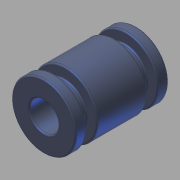
# Autodesk Inventor part: Damper
Saved by Autodesk Inventor 2011 SP2 (Build 150309200, 309)
## iProperties
Created: 2015-02-19
Part Number: Damper
Document SubType Name: Modeling
Designer: Greg Pavlik
Density: 1 g/cm^3
Author: Greg Pavlik
Autodesk Inventor part; units mm, degrees
ref_plane "YZ Plane" through (0, 0, 0) normal (1, 0, 0) x (0, 1, 0)
ref_plane "XZ Plane" through (0, 0, 0) normal (0, 1, 0) x (-1, 0, 0)
ref_plane "XY Plane" through (0, 0, 0) normal (0, 0, 1) x (1, 0, 0)
sketch "Sketch1" plane through (0, 0, 0) normal (0, 0, 1) x (1, 0, 0)
  line L0 (0, 6.5) -> (0, -6.5)
  line L1 (0, 0) -> (-4.5, 0) construction
  line L2 (-2.2, 6.5) -> (-4.3, 6.5)
  line L3 (-4.5, 6.3) -> (-4.5, 5.2)
  line L4 (-4.3, 5) -> (-3.2, 5)
  line L5 (-3, 4.8) -> (-3, 3.7)
  line L6 (-3.2, 3.5) -> (-4.3, 3.5)
  line L7 (-4.5, 3.3) -> (-4.5, -3.3)
  line L8 (-4.3, -3.5) -> (-3.2, -3.5)
  line L9 (-3, -3.7) -> (-3, -4.8)
  line L10 (-3.2, -5) -> (-4.3, -5)
  line L11 (-4.5, -5.2) -> (-4.5, -6.3)
  line L12 (-4.3, -6.5) -> (-2.2, -6.5)
  line L13 (-2, 6.3) -> (-2, -6.3)
  arc A0 (-2, 6.3) -> (-2.2, 6.5) centre (-2.2, 6.3) ccw
  arc A1 (-4.3, 6.5) -> (-4.5, 6.3) centre (-4.3, 6.3) ccw
  arc A2 (-4.5, 5.2) -> (-4.3, 5) centre (-4.3, 5.2) ccw
  arc A3 (-3, 4.8) -> (-3.2, 5) centre (-3.2, 4.8) ccw
  arc A4 (-3.2, 3.5) -> (-3, 3.7) centre (-3.2, 3.7) ccw
  arc A5 (-4.5, -6.3) -> (-4.3, -6.5) centre (-4.3, -6.3) ccw
  arc A6 (-4.3, -5) -> (-4.5, -5.2) centre (-4.3, -5.2) ccw
  arc A7 (-3.2, -5) -> (-3, -4.8) centre (-3.2, -4.8) ccw
  arc A8 (-3, -3.7) -> (-3.2, -3.5) centre (-3.2, -3.7) ccw
  arc A9 (-4.5, -3.3) -> (-4.3, -3.5) centre (-4.3, -3.3) ccw
  arc A10 (-4.3, 3.5) -> (-4.5, 3.3) centre (-4.3, 3.3) ccw
  arc A11 (-2.2, -6.5) -> (-2, -6.3) centre (-2.2, -6.3) ccw
  dimension "d3" = 4
  dimension "d4" = 6
  dimension "d5" = 9
  dimension "d6" = 0.2
  dimension "d8" = 1.5
  dimension "d9" = 13
  dimension "d10" = 3
  constraints: 28 end point, 24 point on circle, 24 tangent, 12 centre point, 11 equal radius, 8 parallel, 3 collinear, 3 perpendicular, 1 midpoint, 1 vertical, 7 other
  measures "d3" diameter of L13 L0
  measures "d4" diameter of L9 L0
  measures "d5" diameter of L11 L0
  measures "d6" radius of A0
  measures "d8" distance between parallel lines of L10 L12
  measures "d9" distance between parallel lines of L2 L12
  measures "d10" distance between parallel lines of L8 L12
revolve "Revolution1" add sketch "Sketch1" angle 360 about axis through (0, 6.5, 0) along (0, -1, 0)
body "Solid1"
